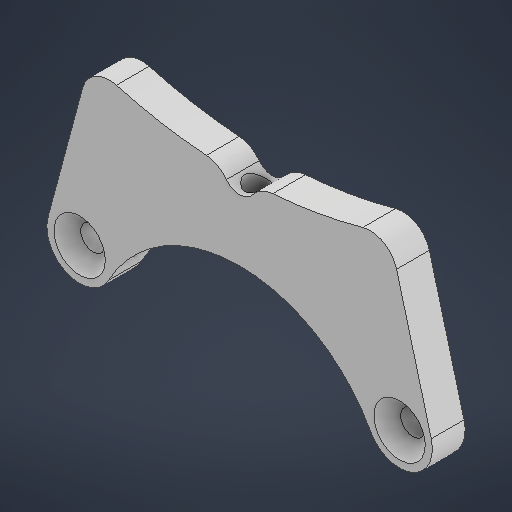
# Autodesk Inventor part: Gradient_positioner
Saved by Autodesk Inventor 2026.1 (Build 301233020, 233B)
## iProperties
Created: 2025-11-19
Part Number: Gradient_positioner
Material: Generic
Document SubType Name: Modeling
Designer: Carla Fernandez
Density: 1 g/cm^3
Appearance: Default
Author: Carla Fernandez
Autodesk Inventor part; units mm, degrees
ref_plane "YZ Plane" through (0, 0, 0) normal (1, 0, 0) x (0, 1, 0)
ref_plane "XY Plane" through (0, 0, 0) normal (0, 0, 1) x (1, 0, 0)
sketch "Sketch1" plane through (0, 0, 0) normal (0, 0, 1) x (1, 0, 0)
  arc A0 (-35.0421, -107.5967) -> (-23.9714, -112.0085) centre (-29.2466, -109.1496) ccw
  arc A1 (-27.3511, -78.8934) -> (27.3511, -78.8934) centre (0, 0) ccw
  line L0 (0, 0) -> (0, -147.6951) construction
  line L1 (0, 0) -> (-29.2466, -109.1496) construction
  line L2 (-35.0421, -107.5967) -> (-27.3511, -78.8934)
  arc A2 (0, -97.7345) -> (-23.9714, -112.0085) centre (0, -125) ccw
  arc A3 (23.9714, -112.0085) -> (35.0421, -107.5967) centre (29.2466, -109.1496) ccw
  line L3 (35.0421, -107.5967) -> (27.3511, -78.8934)
  arc A4 (23.9714, -112.0085) -> (0, -97.7345) centre (0, -125) ccw
  dimension "d0" = 167
  dimension "d1" = 12
  dimension "d2" = 15
  dimension "d3" = 113
  dimension "d4" = 125
  constraints: 12 point on circle, 8 end point, 5 centre point, 5 symmetric about line, 4 point on line, 2 tangent, 1 coincident, 1 parallel, 1 vertical, 2 other
  measures "d0" diameter of A1
  measures "d1" diameter of A0
  measures "d2" angle of L0 L1
  measures "d3" distance of L1.end point (0, 0)
  measures "d4" distance of A2.centre point (0, 0)
extrude "Extrusion1" add sketch "Sketch1" along normal blind 6
sketch "Sketch2" plane through (0, 0, 6) normal (0, 0, 1) x (1, 0, 0)
  line L0 (-29.2466, -109.1496) -> (0, 0) construction
  line L1 (0, 0) -> (29.2466, -109.1496) construction
  line L2 (0, 0) -> (0, -137.2486) construction
  dimension "d14" = 15
  dimension "d15" = 15
  dimension "d16" = 113
  dimension "d17" = 113
  constraints: 6 end point, 1 vertical
  measures "d14" angle of L2 L0
  measures "d15" angle of L1 L2
  measures "d16" distance of L0.start L0.end
  measures "d17" distance of L0.end L1.end
hole "Hole1" at (-29.2466, -109.1496, 6) at (29.2466, -109.1496, 6) direction (0, 0, -1) diameter 4.5 end through all countersink diameter 9.4 countersink angle 90 clearance for "Countersunk Flat Head Screw DIN EN ISO 2009" size "M4" standard "DIN"
fillet "Fillet1" radius 5 2 edges at (-27.3511, -78.8934, 3) (27.3511, -78.8934, 3)
ref_plane "Work Plane1" through (-23.8699, -80.2202, 0) normal (0, 1, 0) x (-1, 0, 0)
sketch "Sketch3" plane through (-23.8699, -80.2202, 0) normal (0, 1, 0) x (-1, 0, 0)
  line L0 (11.1722, 0) -> (11.1722, 6) projected
  point P0 (-23.8699, 0)
  point P1 (-23.8699, 3)
  point P2 (11.1722, 3)
  constraints: 1 horizontal alignment, 1 midpoint, 1 vertical alignment
hole "Hole2" at (0, -80.2202, 3) direction (0, -1, 0) diameter 4 end through all
sketch "Sketch4" plane through (0, 0, 6) normal (0, 0, 1) x (1, 0, 0)
  arc A0 (-22.5214, -80.4055) -> (22.5214, -80.4055) centre (0, 0) ccw projected
  circle A1 centre (0, -83.5) radius 3
  point P0 (0, -83.5)
  point P1 (0, -83.5)
  dimension "d26" = 6
  constraints: 4 point on circle, 2 vertical alignment, 1 centre point
  measures "d26" diameter of A1
extrude "Extrusion2" cut sketch "Sketch4" against normal through all
fillet "Fillet2" radius 5 2 edges at (-2.9995, -83.4461, 3) (2.9995, -83.4461, 3)
equation "\"d15\" = d14"
equation "\"d17\" = d16"
body "Solid1"
